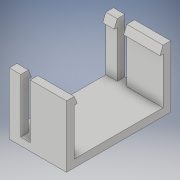
# Autodesk Inventor part: servo clip
Saved by Autodesk Inventor 2019 (Build 230136000, 136)
## iProperties
Created: 2019-01-26
Part Number: servo clip
Material: Generic
Document SubType Name: Modeling
Designer: Brian
Density: 1 g/cm^3
Appearance: Default
Author: Brian
Autodesk Inventor part; units mm, degrees
ref_plane "YZ Plane" through (0, 0, 0) normal (1, 0, 0) x (0, 1, 0)
ref_plane "XZ Plane" through (0, 0, 0) normal (0, 1, 0) x (-1, 0, 0)
ref_plane "XY Plane" through (0, 0, 0) normal (0, 0, 1) x (1, 0, 0)
sketch "Sketch1" plane through (0, 0, 0) normal (0, 1, 0) x (-1, 0, 0)
  line L0 (0, 0) -> (-15, 0)
  line L1 (-15, 0) -> (-15, 27.3)
  line L2 (-15, 27.3) -> (0, 27.3)
  line L3 (0, 27.3) -> (0, 0)
  line L4 (-3, 0) -> (-3, 27.3)
  line L5 (-5.5, 0) -> (-5.5, 27.3)
  line L6 (0, 2) -> (-3, 2)
  line L7 (0, 25.3) -> (-3, 25.3)
  line L8 (-5.5, 2) -> (-15, 2)
  line L9 (-5.5, 25.3) -> (-15, 25.3)
  dimension "d0" = 27.3
  dimension "d1" = 15
  dimension "d2" = 3
  dimension "d3" = 2.5
  dimension "d4" = 2
  dimension "d5" = 2
  dimension "d6" = 2
  dimension "d7" = 2
  constraints: 20 end point, 12 point on line, 7 perpendicular, 2 parallel, 1 horizontal
  measures "d0" distance of L0.end L1.end
  measures "d1" distance of L1.end L2.end
  measures "d2" distance between parallel lines of L3 L4
  measures "d3" distance between parallel lines of L4 L5
  measures "d4" distance between parallel lines of L0 L6
  measures "d5" distance between parallel lines of L2 L7
  measures "d6" distance between parallel lines of L0 L8
  measures "d7" distance between parallel lines of L2 L9
extrude "Extrusion1" add sketch "Sketch1" against normal blind 2
extrude "Extrusion2" add sketch "Sketch1" along normal blind 14.2 contours L0 L4 L6 L3 | L0 L1 L8 L5 | L7 L4 L2 L3 | L9 L1 L2 L5
sketch "Sketch2" plane through (15, -2, 27.3) normal (1, 0, 0) x (0, 0, -1)
  line L0 (25.3, 2) -> (25.3, 16.2) projected
  line L1 (2, 2) -> (2, 16.2) projected
  line L2 (25.3, 16.2) -> (27.3, 16.2) projected
  line L3 (2, 16.2) -> (2.8, 14.2)
  line L4 (2.8, 14.2) -> (2, 14.2)
  line L5 (25.3, 16.2) -> (24.5, 14.2)
  line L6 (24.5, 14.2) -> (25.3, 14.2)
  point P0 (27.3, 2)
  dimension "d12" = 2
  dimension "d13" = 2
  dimension "d14" = 0.8
  dimension "d15" = 0.8
  constraints: 8 end point, 2 point on line, 1 horizontal, 1 perpendicular
  measures "d12" distance from line of L2 L6.end
  measures "d13" distance of L1.end L4.end
  measures "d14" distance of L4.end L3.end
  measures "d15" distance of L5.end L6.end
extrude "Extrusion3" add sketch "Sketch2" against normal up to surface (15 mm away)
sketch "Sketch3" plane through (0, -2, 27.3) normal (0, 0, 1) x (1, 0, 0)
  line L0 (3, 14.2) -> (3, 16.2) projected
  line L1 (5.5, 14.2) -> (3, 14.2) projected
  line L2 (5.5, 14.2) -> (5.5, 16.2) projected
  line L3 (5.5, 16.2) -> (3, 16.2) projected
  point P0 (0, 2)
extrude "Extrusion4" cut sketch "Sketch3" against normal through all
body "Solid1"
